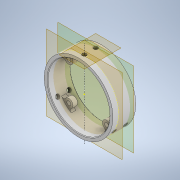
# Autodesk Inventor part: Verbindungsring
Saved by Autodesk Inventor 2020 (Build 240168000, 168)
## iProperties
Created: 2022-02-05
Part Number: Verbindungsring
Material: Generisch
Document SubType Name: Modeling
Designer: sp
Density: 1 g/cm^3
Appearance: Vorgabe
Author: sp
## iProperties of the stored document _3D-Druck.ipt
Created: 2022-05-02
Part Number: _3D-Druck
Material: Generisch
Document SubType Name: Modeling
Designer: sp
Density: 1 g/cm^3
Appearance: Vorgabe
Author: sp
Autodesk Inventor part; units mm, degrees
ref_plane "YZ Plane" through (0, 0, 0) normal (1, 0, 0) x (0, 1, 0)
ref_plane "XZ Plane" through (0, 0, 0) normal (0, 1, 0) x (-1, 0, 0)
sketch "Skizze1" plane through (0, 0, 0) normal (0, 0, 1) x (1, 0, 0)
  circle A0 centre (0, 0) radius 30
  circle A1 centre (0, 0) radius 27
  dimension "d0" = 60
  dimension "d1" = 54
  constraints: 2 centre point, 2 coincident
  measures "d0" diameter of A0
  measures "d1" diameter of A1
extrude "Extrusion1" add sketch "Skizze1" along normal mid plane 20
ref_plane "Arbeitsebene1" through (0, 0, 5) normal (0, 0, 1) x (1, 0, 0)
sketch "Skizze2" plane through (0, 0, 5) normal (0, 0, 1) x (1, 0, 0)
  line L0 (0, 39.0372) -> (0, -37.5893) construction
  circle A0 centre (0, 0) radius 30 construction
  point P0 (0, 30)
  constraints: 2 end point, 2 point on line, 1 vertical, 1 vertical alignment, 1 other
ref_plane "Arbeitsebene2" through (0, 30, 5) normal (0, 1, 0) x (-1, 0, 0)
sketch "Skizze3" plane through (0, 30, 5) normal (0, 1, 0) x (-1, 0, 0)
  circle A0 centre (0, 0) radius 1.75
  point P0 (0, -5)
  dimension "d5" = 3.5
  constraints: 1 centre point
  measures "d5" diameter of A0
extrude "Extrusion2" cut sketch "Skizze3" against normal blind 5
pattern_circular "Runde Anordnung1" count 3 over 360 about axis through (0, 0, -10) along (0, 0, 1) of "Extrusion2"
mirror "Spiegeln1" about plane through (0, 0, 0) normal (0, 0, 1) of "Extrusion2", "Runde Anordnung1"
chamfer "Fase1" distance 0.5 angle 45 2 edges at (-27, 0, 10) (-27, 0, -10)
sketch "Skizze4" plane through (0, 0, 0) normal (0, 0, 1) x (1, 0, 0)
  line L0 (0, 34.5644) -> (0, -38.5024) construction
  line L1 (-38.0901, 0) -> (52.3904, 0) construction
  line L2 (-34.7368, 16.5) -> (36.624, 16.5) construction
  line L3 (-36.0898, -16.5) -> (37.8594, -16.5) construction
  line L4 (16.5, 35.2115) -> (16.5, -32.6782) construction
  line L5 (-16.5, 34.5644) -> (-16.5, -34.6196) construction
  circle A0 centre (-16.5, 16.5) radius 1.75
  circle A1 centre (16.5, 16.5) radius 1.75
  circle A2 centre (-16.5, -16.5) radius 1.75
  circle A3 centre (16.5, -16.5) radius 1.75
  circle A4 centre (-16.5, 16.5) radius 3.6693
  circle A5 centre (16.5, 16.5) radius 3.7169
  circle A6 centre (16.5, -16.5) radius 3.6667
  circle A7 centre (-16.5, -16.5) radius 3.6675
  point P0 (0, 0)
  dimension "d14" = 33
  dimension "d15" = 33
  dimension "d16" = 3.5
  dimension "d17" = 3.5
  dimension "d18" = 3.5
  dimension "d19" = 3.5
  constraints: 12 end point, 10 point on line, 8 centre point, 4 coincident, 3 horizontal, 3 vertical, 2 other
  measures "d14" distance between parallel lines of L3 L2
  measures "d15" distance between parallel lines of L5 L4
  measures "d16" diameter of A0
  measures "d17" diameter of A1
  measures "d18" diameter of A2
  measures "d19" diameter of A3
extrude "Extrusion3" add sketch "Skizze4" along normal mid plane 4
fillet "Rundung1" radius 2 14 edges at (-19.2192, 18.9637, 1) (-19.2192, 18.9637, -1) (-18.9637, 19.2192, -1) (-18.9637, 19.2192, 1) (19.5548, 18.6175, 0) (18.6175, 19.5548, 0) (19.1626, -19.0209, 1) (19.1626, -19.0209, -1) (19.0209, -19.1626, -1) (19.0209, -19.1626, 1) (-18.9987, -19.1846, 1) (-18.9987, -19.1846, -1) (-19.1846, -18.9987, -1) (-19.1846, -18.9987, 1)
ref_plane "Arbeitsebene3" through (0, 0, -5) normal (0, 0, 1) x (1, 0, 0)
ref_plane "Arbeitsebene4" through (0, 30, -5) normal (0, -1, 0) x (-1, 0, 0)
